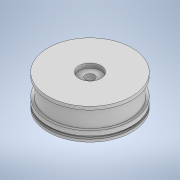
# Autodesk Inventor part: Нижняя часть поршня
Saved by Autodesk Inventor 2021 (Build 250183000, 183)
## iProperties
Created: 2020-10-24
Part Number: Нижняя часть поршня
Material: Типовые
Document SubType Name: Modeling
Designer: Тимоха
Density: 1 g/cm^3
Appearance: По умолчанию
Author: Тимоха
Autodesk Inventor part; units mm, degrees
ref_plane "YZ Plane" through (0, 0, 0) normal (1, 0, 0) x (0, 1, 0)
ref_plane "XZ Plane" through (0, 0, 0) normal (0, 1, 0) x (-1, 0, 0)
ref_plane "XY Plane" through (0, 0, 0) normal (0, 0, 1) x (1, 0, 0)
sketch "Эскиз1" plane through (0, 0, 0) normal (0, 0, 1) x (1, 0, 0)
  line L0 (49.9998, 0) -> (189, 0)
  line L1 (189, 0) -> (189, -15)
  line L2 (189, -15) -> (178, -15)
  line L3 (178, -15) -> (178, -95)
  line L4 (178, -95) -> (189, -95)
  line L5 (137.0508, -39) -> (70.9998, -39)
  line L6 (24.9998, -84) -> (19.9998, -84)
  line L7 (19.9998, -84) -> (19.9998, -20)
  line L8 (19.9998, -20) -> (49.9998, -20)
  line L9 (49.9998, -20) -> (49.9998, 0)
  arc A0 (70.9998, -39) -> (54.9998, -55) centre (70.9998, -55) ccw
  arc A1 (152.99, -56.3945) -> (137.0508, -39) centre (137.0508, -55) ccw
  arc A2 (34.9998, -94) -> (24.9998, -84) centre (24.9998, -94) ccw
  line L10 (0, 0) -> (0, 25.6698)
  line L11 (189, -95) -> (189, -116)
  line L12 (189, -140) -> (169, -140)
  line L13 (189, -140) -> (189, -128)
  line L14 (189, -128) -> (178, -128)
  line L15 (178, -128) -> (178, -116)
  line L16 (178, -116) -> (189, -116)
  line L17 (189, -95) -> (189, -116)
  line L18 (34.9998, -140) -> (34.9998, -94)
  line L19 (39.9998, -140) -> (34.9998, -140)
  line L20 (169, -140) -> (169, -132)
  line L21 (169, -132) -> (149, -132)
  line L22 (149, -132) -> (149, -86)
  line L23 (149, -86) -> (152.99, -56.3945)
  line L24 (39.9998, -140) -> (39.9998, -132)
  line L25 (39.9998, -132) -> (54.9998, -132)
  line L26 (54.9998, -132) -> (54.9998, -55)
  point P0 (154.5118, -39)
  point P1 (54.9998, -39)
  point P2 (34.9998, -84)
  dimension "d0" = 189
  dimension "d1" = 15
  dimension "d2" = 11
  dimension "d3" = 80
  dimension "d5" = 99.512
  dimension "d6" = 15
  dimension "d7" = 64
  dimension "d8" = 30
  dimension "d9" = 16
  dimension "d10" = 16
  dimension "d11" = 10
  dimension "d12" = 20
  dimension "d14" = 12
  dimension "d15" = 11
  dimension "d16" = 12
  dimension "d17" = 21
  dimension "d20" = 46
  dimension "d22" = 8
  dimension "d23" = 46
  constraints: 54 end point, 11 perpendicular, 7 vertical, 6 point on circle, 4 point on line, 3 centre point, 3 tangent, 2 horizontal, 1 collinear
  measures "d0" distance of L10.start L0.end
  measures "d1" distance of L0.end L2.start
  measures "d2" distance of L2.start L3.start
  measures "d3" distance of L3.start L3.end
  measures "d5" distance of point (154.512, -39) point (55, -39)
  measures "d6" distance of point (35, -84) L7.start
  measures "d7" distance of L7.start L7.end
  measures "d8" distance of L7.end L8.end
  measures "d9" radius of A0
  measures "d10" radius of A1
  measures "d11" radius of A2
  measures "d12" distance of L12.start L12.end
  measures "d14" distance of L14.start L12.start
  measures "d15" distance of L14.start L15.start
  measures "d16" distance of L15.start L15.end
  measures "d17" distance of L4.end L11.end
  measures "d20" distance of L18.start L18.end
  measures "d22" distance of L12.end L20.end
  measures "d23" distance of L21.end L22.end
revolve "Вращение1" add sketch "Эскиз1" angle 360 about axis through (0, 0, 0) along (0, 1, 0)
